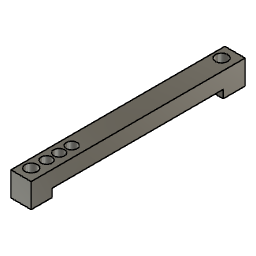
Fiberoptic holder (Autodesk Fusion 360 design; units mm, degrees)
Autodesk Fusion 360 part; units mm, degrees
note: some values were not read from the file. Set by a fixed rule: which face or edge a step refers to.
sketch "Sketch1" plane through (0, 0, 0) normal (0, 0, 1) x (1, 0, 0)
  circle A0 centre (0, 0) radius 1.5
  line L0 (2.9, 0) -> (2.9, -2.9)
  line L1 (2.9, -2.9) -> (0, -2.9)
  circle A1 centre (0, 47) radius 1.5
  line L2 (0, 49.9) -> (2.9, 49.9)
  line L3 (2.9, 49.9) -> (2.9, 47)
  line L4 (2.9, -2.9) -> (-2.1, -2.9)
  line L5 (-2.1, -2.9) -> (-2.1, 49.9)
  line L6 (-2.1, 49.9) -> (2.9, 49.9)
  line L7 (2.9, 49.9) -> (2.9, -2.9)
  line L8 (1.3, 4.05) -> (0.1, 4.05)
  line L9 (0.1, 4.05) -> (0.1, 3.15)
  line L10 (0.1, 3.15) -> (1.3, 3.15)
  line L11 (1.3, 3.15) -> (1.3, 4.05)
  line L12 (1.3, 4.05) -> (0.1, 3.15) construction
  line L13 (0.1, 4.05) -> (1.3, 3.15) construction
  line L14 (1.3, 7.1) -> (0.1, 7.1)
  line L15 (0.1, 7.1) -> (0.1, 6.3)
  line L16 (0.1, 6.3) -> (1.3, 6.3)
  line L17 (1.3, 6.3) -> (1.3, 7.1)
  line L18 (1.3, 7.1) -> (0.1, 6.3) construction
  line L19 (0.1, 7.1) -> (1.3, 6.3) construction
  line L20 (1.3, 10.2) -> (0.1, 10.2)
  line L21 (0.1, 10.2) -> (0.1, 9.4)
  line L22 (0.1, 9.4) -> (1.3, 9.4)
  line L23 (1.3, 9.4) -> (1.3, 10.2)
  line L24 (1.3, 10.2) -> (0.1, 9.4) construction
  line L25 (0.1, 10.2) -> (1.3, 9.4) construction
  circle A2 centre (0.7, 3.6) radius 1.075
  circle A3 centre (0.7, 6.7) radius 1.075
  circle A4 centre (0.7, 9.8) radius 1.075
  line L26 (0.7, 2.525) -> (-2.1, 2.525)
  line L27 (0.7, 2.525) -> (2.9, 2.525)
  line L28 (0, 45.5) -> (0, 44.5)
  line L29 (0, 44.5) -> (-2.1, 44.5)
  line L30 (0, 44.5) -> (2.9, 44.5)
  line L31 (2.9, 3.6) -> (1.3, 3.6)
  point P0 (0.7, 3.6)
  point P1 (0.7, 6.7)
  point P2 (0.7, 9.8)
  dimension "d1" = 3
  dimension "d5" = 3
  dimension "d8" = 5
  dimension "d22" = 1
  dimension "d23" = 1.6
  constraint coincident A0.centre origin
  constraint perpendicular L0 L1
  constraint horizontal L4
  constraint vertical L5
  constraint horizontal L6
  constraint vertical L7
  constraint horizontal L8
  constraint perpendicular L8 L9
  constraint parallel L8 L10
  constraint parallel L9 L11
  constraint coincident L12 P0
  constraint coincident L13 P0
  constraint horizontal L14
  constraint perpendicular L14 L15
  constraint parallel L14 L16
  constraint parallel L15 L17
  constraint coincident L18 P1
  constraint coincident L19 P1
  constraint horizontal L20
  constraint perpendicular L20 L21
  constraint parallel L20 L22
  constraint parallel L21 L23
  constraint coincident L24 P2
  constraint coincident L25 P2
  constraint coincident P0 A2.centre
  constraint coincident P1 A3.centre
  constraint coincident P2 A4.centre
  constraint coincident A2 L26.start
  constraint coincident L5 L26.end
  constraint tangent A2 L26
  constraint perpendicular L5 L26
  constraint coincident L7 L27.end
  constraint tangent A2 L27
  constraint coincident A1 L28.start
  constraint perpendicular L27 L28
  constraint coincident L5 L29.end
  constraint perpendicular L5 L29
  constraint coincident L7 L30.end
  constraint perpendicular L7 L30
  constraint coincident L7 L31.start
  constraint perpendicular L7 L31
  measures "d1" diameter of A0
  measures "d5" diameter of A1
  measures "d8" distance of L0.end L4.end
  measures "d22" distance of L28.start L28.end
  measures "d23" distance of L31.start L31.end
extrude "Extrude1" add sketch "Sketch1" against normal blind 2 contours L0 L1 L4 L5 L7 L26 L27 | L2 L3 L5 L6 L7 L29 L30 makes body 1 at (2.4333, -0.125, 0) makes body 2 at (2.4333, 47.1333, -2)
extrude "Extrude2" add sketch "Sketch1" along normal blind 4 contours L0 L1 L4 L5 L7 L26 L27 | L7 A2 L27 L31 | L5 L7 A2 L26 L29 L30 L31 | L2 L3 L5 L6 L7 L29 L30 bodies 1 2
move_face "MoveFace1" to x (1, 0, 0) y (0, 1, 0) z (0, 0, 1) at (-0.5, 0, 0) 4 faces at (-0.2221, 4.1527, 2.6667) (1.7738, 3.5488, 2.6667) (1.7737, 6.6464, 2.6667) (1.7737, 9.7464, 2.6667) on bodies 1
move_face "OffsetFaces1" offset -0.1 3 faces at (0.2, 2.525, 2.6667) (1.2737, 6.6464, 2.6667) (1.2737, 9.7464, 2.6667) on bodies 1
move_face "OffsetFaces2" offset -0.15 3 faces at (0.2, 2.425, 2.6667) (1.3735, 6.6414, 2.6667) (1.3735, 9.7414, 2.6667) on bodies 1
extrude "Extrude3" cut 6 faces at (0.7424, 2.4469, 0) (0.2541, 2.4621, 0) (0.1459, 2.4621, 0) (-0.3424, 2.4469, 0) (-0.0889, 2.361, 0) (0.6062, 2.3944, 0) along direction (0, 0, -1) blind 32.5 on bodies 1 bodies 1
sketch "Sketch2" plane through (0, 0, -2) normal (0, 0, -1) x (1, 0, 0)
  arc A0 (0.9746, -2.525) -> (-0.5746, -2.525) centre (0.2, -3.6) ccw
  line L0 (0.9746, -2.525) -> (2.9, -2.525)
  line L1 (2.9, -2.525) -> (2.9, 2.9)
  line L2 (2.9, 2.9) -> (-2.1, 2.9)
  line L3 (-2.1, 2.9) -> (-2.1, -2.525)
  line L4 (-2.1, -2.525) -> (-0.5746, -2.525)
  circle A1 centre (0, 0) radius 1.5
  line L5 (0.2, -2.275) -> (-2.1, -2.275)
  line L6 (0.2, -2.275) -> (2.9, -2.275)
  constraint midpoint A0 L5.start
  constraint coincident L3 L5.end
  constraint tangent A0 L5
  constraint perpendicular L3 L5
  constraint coincident L1 L6.end
  constraint tangent A0 L6
  constraint perpendicular L1 L6
extrude "Extrude4" cut sketch "Sketch2" against normal blind 2 contours A0 L0 L1 L6 | A0 L3 L4 L5 bodies 1
equation "d29 = ( -0.3 / 2 ) * 1 mm"
